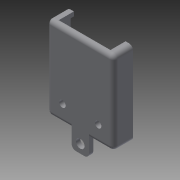
# Autodesk Inventor part: bottom
Saved by Autodesk Inventor 2014 SP1 (Build 180222100, 222)
## iProperties
Created: 2016-10-19
Part Number: bottom
Material: Generic
Document SubType Name: Modeling
Designer: danielsikar
Density: 1 g/cm^3
Appearance: Default
Author: danielsikar
Autodesk Inventor part; units mm, degrees
ref_plane "YZ Plane" through (0, 0, 0) normal (1, 0, 0) x (0, 1, 0)
ref_plane "XZ Plane" through (0, 0, 0) normal (0, 1, 0) x (-1, 0, 0)
ref_plane "XY Plane" through (0, 0, 0) normal (0, 0, 1) x (1, 0, 0)
sketch "Sketch1" plane through (0, 0, 0) normal (0, 1, 0) x (-1, 0, 0)
  line L0 (0, 0) -> (30.9, 0)
  line L1 (30.9, 0) -> (30.9, 38.5)
  line L2 (30.9, 38.5) -> (0, 38.5)
  line L3 (0, 38.5) -> (0, 0)
  dimension "d0" = 30.9
  dimension "d1" = 38.5
  constraints: 8 end point, 2 parallel, 1 horizontal, 1 perpendicular
  measures "d0" distance of L2.end L1.end
  measures "d1" distance between parallel lines of L0 L2
extrude "Extrusion1" add sketch "Sketch1" along normal blind 2
sketch "Sketch2" plane through (0, 2, 0) normal (0, 1, 0) x (1, 0, 0)
  line L0 (-30.9, 0) -> (-30.9, -38.5) projected
  line L1 (-30.9, -38.5) -> (0, -38.5) projected
  circle A0 centre (-23.7, -7.8) radius 3
  circle A1 centre (-7.2, -7.8) radius 3
  dimension "d4" = 6
  dimension "d5" = 6
  dimension "d6" = 30.7
  dimension "d7" = 30.7
  dimension "d8" = 7.2
  dimension "d9" = 16.5
  constraints: 2 centre point
  measures "d4" diameter of A0
  measures "d5" diameter of A1
  measures "d6" distance from line of L1 A0.centre
  measures "d7" distance from line of L1 A1.centre
  measures "d8" distance from line of A0.centre L0
  measures "d9" distance of A1.centre A0.centre
extrude "Extrusion2" add sketch "Sketch2" along normal blind 7
sketch "Sketch3" plane through (-23.7, 9, 7.8) normal (0, 1, 0) x (1, 0, 0)
  circle A0 centre (0, 0) radius 3 projected
  circle A1 centre (0, 0) radius 1.5
  point P0 (23.7, 7.8)
  dimension "d12" = 3
  constraints: 1 centre point, 1 coincident
  measures "d12" diameter of A1
extrude "Extrusion3" cut sketch "Sketch3" against normal blind 9 contours A1
sketch "Sketch4" plane through (-7.2, 9, 7.8) normal (0, 1, 0) x (1, 0, 0)
  circle A0 centre (0, 0) radius 3 projected
  circle A1 centre (0, 0) radius 1.5
  point P0 (7.2, 7.8)
  dimension "d15" = 3
  constraints: 1 centre point, 1 coincident
  measures "d15" diameter of A1
extrude "Extrusion4" cut sketch "Sketch4" against normal blind 10 contours A1
sketch "Sketch5" plane through (0, 2, 0) normal (0, 1, 0) x (1, 0, 0)
  line L0 (-30.9, 0) -> (-30.9, -38.5) projected
  line L1 (-30.9, -38.5) -> (0, -38.5) projected
  line L2 (-30.9, 0) -> (0, 0)
  line L3 (0, 0) -> (0, -38.5)
  line L4 (0, -38.5) -> (-30.9, -38.5)
  line L5 (-30.9, -38.5) -> (-30.9, 0)
  line L6 (-28.9, -2) -> (-2, -2)
  line L7 (-2, -2) -> (-2, -36.5)
  line L8 (-2, -36.5) -> (-28.9, -36.5)
  line L9 (-28.9, -36.5) -> (-28.9, -2)
  dimension "d18" = 26.9
  dimension "d19" = 34.5
  dimension "d20" = 2
  dimension "d21" = 2
  constraints: 16 end point, 4 parallel, 2 horizontal, 2 perpendicular
  measures "d18" distance of L7.end L8.end
  measures "d19" distance of L6.end L7.end
  measures "d20" distance between parallel lines of L1 L8
  measures "d21" distance between parallel lines of L9 L0
extrude "Extrusion5" add sketch "Sketch5" along normal blind 7
sketch "Sketch6" plane through (-30.9, 0, 38.5) normal (0, 0, 1) x (1, 0, 0)
  line L0 (0, 9) -> (30.9, 9) projected
  line L1 (0, 0) -> (0, 9) projected
  line L2 (3.5, 9) -> (27.4, 9)
  line L3 (27.4, 9) -> (27.4, -6)
  line L4 (27.4, -6) -> (3.5, -6)
  line L5 (3.5, -6) -> (3.5, 9)
  dimension "d24" = 23.9
  dimension "d25" = 15
  dimension "d26" = 3.5
  constraints: 8 end point, 2 parallel, 1 horizontal, 1 perpendicular, 1 point on line
  measures "d24" distance of L3.end L4.end
  measures "d25" distance of L2.end L3.end
  measures "d26" distance between parallel lines of L5 L1
extrude "Extrusion6" cut sketch "Sketch6" against normal blind 2
fillet "Fillet1" radius 2 9 edges at (0, 4.5, 38.5) (-30.9, 4.5, 38.5) (0, 4.5, 0) (-30.9, 4.5, 0) (-1.75, 0, 38.5) (-29.15, 0, 38.5) (-30.9, 0, 19.25) (0, 0, 19.25) (-15.45, 0, 0)
sketch "Sketch7" plane through (-2, 0, 0) normal (0, 0, -1) x (-1, 0, 0)
  line L0 (0, 0) -> (26.9, 0) projected
  line L1 (9.45, 0) -> (17.45, 0)
  line L2 (17.45, 0) -> (17.45, 2)
  line L3 (17.45, 2) -> (9.45, 2)
  line L4 (9.45, 2) -> (9.45, 0)
  line L5 (-2, 9) -> (-2, 2) projected
  point P0 (-2, 0)
  dimension "d30" = 8
  dimension "d31" = 2
  dimension "d32" = 11.45
  constraints: 8 end point, 2 parallel, 1 horizontal, 1 perpendicular, 1 point on line
  measures "d30" distance of L3.end L2.end
  measures "d31" distance of L2.end L1.end
  measures "d32" distance between parallel lines of L4 L5
extrude "Extrusion7" add sketch "Sketch7" along normal blind 8
sketch "Sketch8" plane through (-19.45, 2, 0) normal (0, 1, 0) x (1, 0, 0)
  circle A0 centre (4, 4) radius 2
  point P0 (19.45, 0)
  dimension "d35" = 4
  constraints: 1 centre point
  measures "d35" diameter of A0
extrude "Extrusion8" cut sketch "Sketch8" against normal up to next
fillet "Fillet2" radius 2 2 edges at (-11.45, 1, -8) (-19.45, 1, -8)
sketch "Sketch9" plane through (-2, 0, 0) normal (0, 0, 1) x (1, 0, 0)
  line L0 (-9.45, 0) -> (-17.45, 0) projected
  line L1 (-9.45, 2) -> (-9.45, 0) projected
  line L2 (-17.45, 0) -> (-9.45, 0)
  line L3 (-9.45, 0) -> (-9.45, 2)
  line L4 (-9.45, 2) -> (-17.45, 2)
  line L5 (-17.45, 2) -> (-17.45, 0)
  point P0 (2, 0)
  constraints: 8 end point, 2 parallel, 1 horizontal, 1 perpendicular
extrude "Extrusion9" add sketch "Sketch9" along normal blind 8
sketch "Sketch11" plane through (-30.9, 0, 36.5) normal (0, 0, 1) x (1, 0, 0)
  line L0 (27.4, 0) -> (3.5, 0) projected
  line L1 (27.4, 2) -> (27.4, 0) projected
  line L2 (27.4, 2) -> (3.5, 2)
  line L3 (3.5, 2) -> (3.5, 0)
  line L4 (3.5, 0) -> (27.4, 0)
  line L5 (27.4, 0) -> (27.4, 2)
  point P0 (30.9, 0)
  constraints: 8 end point, 2 parallel, 1 horizontal, 1 perpendicular
extrude "Extrusion12" add sketch "Sketch11" along normal blind 2
fillet "Fillet3" radius 2 1 edges at (-15.45, 0, 38.5)
body "Solid1"
